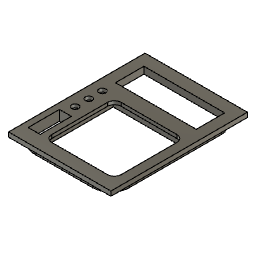
Ferdinant_Deckel v1 (Autodesk Fusion 360 design; units mm, degrees)
Autodesk Fusion 360 part; units mm, degrees
sketch "Skizze1" plane through (0, 0, 0) normal (0, 0, 1) x (1, 0, 0)
  line L0 (-52.263, 59.6389) -> (37.737, 59.6389)
  line L1 (37.737, 59.6389) -> (37.737, -60.3611)
  line L2 (37.737, -60.3611) -> (-52.263, -60.3611)
  line L3 (-52.263, -60.3611) -> (-52.263, 59.6389)
  dimension "d1" = 90
  dimension "d2" = 120
  constraint horizontal L0
  constraint vertical L1
  constraint horizontal L2
  constraint vertical L3
  measures "d1" distance of L0.start L0.end
  measures "d2" distance of L0.end L1.end
extrude "Extrusion1" add sketch "Skizze1" against normal blind 3
extrude "Extrusion2" add 1 faces at (-22.263, 19.6389, 0) along direction (0, 0, 1) blind 1
sketch "Skizze2" plane through (0, 0, 1) normal (0, 0, 1) x (-1, 0, 0)
  line L0 (52.263, 60.3611) -> (-37.737, 60.3611)
  line L1 (-37.737, 60.3611) -> (-37.737, -59.6389)
  line L2 (-37.737, -59.6389) -> (52.263, -59.6389)
  line L3 (52.263, -59.6389) -> (52.263, 60.3611)
  line L4 (25.263, -11.6389) -> (-23.737, -11.6389)
  line L5 (-29.737, -5.6389) -> (-29.737, 43.3611)
  line L6 (-23.737, 49.3611) -> (25.263, 49.3611)
  line L7 (31.263, 43.3611) -> (31.263, -5.6389)
  line L8 (33.263, -12.6389) -> (-31.737, -12.6389)
  line L9 (-31.737, -12.6389) -> (-31.737, 52.3611)
  line L10 (-31.737, 52.3611) -> (33.263, 52.3611)
  line L11 (33.263, 52.3611) -> (33.263, -12.6389)
  line L12 (42.763, -49.1389) -> (-28.237, -49.1389)
  line L13 (-28.237, -49.1389) -> (-28.237, -24.1389)
  line L14 (-28.237, -24.1389) -> (42.763, -24.1389)
  line L15 (42.763, -24.1389) -> (42.763, -49.1389)
  circle A0 centre (42.263, -12.1389) radius 3
  circle A1 centre (42.263, -0.1389) radius 3
  circle A2 centre (42.263, 11.8611) radius 3
  line L16 (47.013, 20.8611) -> (36.513, 20.8611)
  line L17 (36.513, 20.8611) -> (36.513, 48.3611)
  line L18 (36.513, 48.3611) -> (47.013, 48.3611)
  line L19 (47.013, 48.3611) -> (47.013, 20.8611)
  arc A3 (-29.737, -5.6389) -> (-23.737, -11.6389) centre (-23.737, -5.6389) ccw
  arc A4 (25.263, -11.6389) -> (31.263, -5.6389) centre (25.263, -5.6389) ccw
  arc A5 (31.263, 43.3611) -> (25.263, 49.3611) centre (25.263, 43.3611) ccw
  arc A6 (-23.737, 49.3611) -> (-29.737, 43.3611) centre (-23.737, 43.3611) ccw
  point P0 (31.263, -11.6389)
  point P1 (-29.737, -11.6389)
  point P2 (31.263, 49.3611)
  dimension "d7" = 61
  dimension "d8" = 61
  dimension "d10" = 11
  dimension "d11" = 65
  dimension "d12" = 65
  dimension "d13" = 8
  dimension "d19" = 25
  dimension "d20" = 71
  dimension "d23" = 8
  dimension "d24" = 6
  dimension "d25" = 6
  dimension "d26" = 9
  dimension "d28" = 6
  dimension "d29" = 6
  dimension "d30" = 12
  dimension "d31" = 9
  dimension "d32" = 9
  dimension "d33" = 12
  dimension "d34" = 10.5
  dimension "d35" = 27.5
  dimension "d36" = 12
  dimension "d37" = 5.25
  dimension "d62" = 6
  dimension "d63" = 6
  dimension "d82" = 12
  constraint horizontal L4
  constraint vertical L5
  constraint horizontal L6
  constraint vertical L7
  constraint horizontal L8
  constraint vertical L9
  constraint horizontal L10
  constraint vertical L11
  constraint horizontal L12
  constraint vertical L13
  constraint horizontal L14
  constraint vertical L15
  constraint horizontal L16
  constraint vertical L17
  constraint horizontal L18
  constraint vertical L19
  constraint coincident P1 L4
  constraint coincident P1 L5
  constraint tangent L4 A3
  constraint tangent L5 A3
  constraint coincident P0 L4
  constraint coincident P0 L7
  constraint tangent L4 A4
  constraint tangent L7 A4
  constraint coincident P2 L6
  constraint coincident P2 L7
  constraint tangent L6 A5
  constraint tangent L7 A5
  constraint equal A4 A5
  constraint tangent L5 A6
  constraint tangent L6 A6
  constraint equal A4 A6
  measures "d7" distance of P0 P1
  measures "d8" distance of P0 P2
  measures "d10" distance of L0 L6
  measures "d11" distance of L8.start L8.end
  measures "d12" distance of L8.start L10.end
  measures "d13" distance of L0 L10
  measures "d19" distance of L12.start L14.end
  measures "d20" distance of L12.start L12.end
  measures "d23" distance of L1 L5
  measures "d24" distance of L1 L9
  measures "d25" diameter of A0
  measures "d26" distance of L11 A0.centre
  measures "d28" diameter of A1
  measures "d29" diameter of A2
  measures "d30" vertical distance of A0.centre A1.centre
  measures "d31" distance of L11 A1.centre
  measures "d32" distance of L11 A2.centre
  measures "d33" distance of A1.centre A2.centre
  measures "d34" distance of L16.start L16.end
  measures "d35" distance of L16.start L18.end
  measures "d36" distance of L0 L18
  measures "d37" distance of L3 L19
  measures "d62" radius of A3
  measures "d63" radius of A4
  measures "d82" distance of L14 A0.centre
sketch "Skizze3" plane through (0, 0, -3) normal (0, 0, -1) x (1, 0, 0)
  line L0 (37.737, 60.3611) -> (-52.263, 60.3611)
  line L1 (-52.263, 60.3611) -> (-52.263, -59.6389)
  line L2 (-52.263, -59.6389) -> (37.737, -59.6389)
  line L3 (37.737, -59.6389) -> (37.737, 60.3611)
  line L4 (-32.763, 56.8611) -> (18.237, 56.8611)
  line L5 (34.237, 40.8611) -> (34.237, -56.1389)
  line L6 (34.237, -56.1389) -> (-48.763, -56.1389)
  line L7 (-48.763, -56.1389) -> (-48.763, 40.8611)
  arc A0 (34.237, 40.8611) -> (18.237, 56.8611) centre (18.237, 40.8611) ccw
  arc A1 (-32.763, 56.8611) -> (-48.763, 40.8611) centre (-32.763, 40.8611) ccw
  line L8 (-52.263, 0.3611) -> (37.737, 0.3611)
  arc A2 (-48.763, -40.1389) -> (-32.763, -56.1389) centre (-32.763, -40.1389) ccw
  arc A3 (18.237, -56.1389) -> (34.237, -40.1389) centre (18.237, -40.1389) ccw
  dimension "d38" = 3.5
  dimension "d39" = 3.5
  dimension "d40" = 3.5
  dimension "d41" = 3.5
  dimension "d45" = 16
  dimension "d46" = 16
  constraint horizontal L4
  constraint vertical L5
  constraint horizontal L6
  constraint vertical L7
  constraint tangent L4 A0
  constraint tangent L5 A0
  constraint tangent L4 A1
  constraint tangent L7 A1
  constraint midpoint L1 L8.start
  constraint midpoint L3 L8.end
  constraint symmetric L4.end L8 A3.start
  constraint symmetric L5.start L8 A3.end
  constraint symmetric A0 L8 A3
  constraint symmetric L4.start L8 A2.end
  constraint symmetric L7.end L8 A2.start
  constraint symmetric A1 L8 A2
  measures "d38" distance of L1 L7
  measures "d39" distance of L3 L5
  measures "d40" distance of L0 L4
  measures "d41" distance of L2 L6
  measures "d45" radius of A0
  measures "d46" radius of A1
extrude "Extrusion3" add sketch "Skizze3" along normal blind 5 contours L4 L5 L7 A0 A1 L8 | L5 L6 L7 L8 A2 A3
extrude "Extrusion4" cut sketch "Skizze2" against normal blind 9 contours A1
extrude "Extrusion5" cut sketch "Skizze2" against normal blind 9 contours A0 | A2
sketch "Skizze4" plane through (0, 0, -8) normal (0, 0, -1) x (1, 0, 0)
  circle A0 centre (-42.263, -12.1389) radius 3
  circle A1 centre (-42.263, 11.8611) radius 3
  circle A2 centre (-42.263, -0.1389) radius 3
  arc A3 (-48.763, -40.1389) -> (-32.763, -56.1389) centre (-32.763, -40.1389) ccw
  line L0 (-32.763, -56.1389) -> (18.237, -56.1389)
  arc A4 (18.237, -56.1389) -> (34.237, -40.1389) centre (18.237, -40.1389) ccw
  line L1 (34.237, -40.1389) -> (34.237, 40.8611)
  arc A5 (34.237, 40.8611) -> (18.237, 56.8611) centre (18.237, 40.8611) ccw
  line L2 (18.237, 56.8611) -> (-32.763, 56.8611)
  arc A6 (-32.763, 56.8611) -> (-48.763, 40.8611) centre (-32.763, 40.8611) ccw
  line L3 (-48.763, 40.8611) -> (-48.763, -40.1389)
  circle A7 centre (-42.263, 11.8611) radius 4
  circle A8 centre (-42.263, -0.1389) radius 4
  circle A9 centre (-42.263, -12.1389) radius 4
  dimension "d53" = 8
  dimension "d54" = 8
  dimension "d55" = 8
  constraint concentric A1 A7
  constraint concentric A2 A8
  constraint concentric A0 A9
  measures "d53" diameter of A7
  measures "d54" diameter of A8
  measures "d55" diameter of A9
extrude "Extrusion6" cut sketch "Skizze4" against normal blind 6 contours A7 | A8 | A9
extrude "Extrusion7" cut sketch "Skizze2" against normal blind 9 contours L16 L17 L18 L19
extrude "Extrusion8" cut sketch "Skizze2" against normal blind 9 contours L12 L13 L14 L15
extrude "Extrusion9" cut sketch "Skizze2" against normal blind 9 contours L4 L5 L6 L7 A3 A4 A5 A6
sketch "Skizze5" plane through (0, 0, -8) normal (0, 0, -1) x (1, 0, 0)
  line L0 (-25.263, 49.3611) -> (23.737, 49.3611)
  arc A0 (29.737, 43.3611) -> (23.737, 49.3611) centre (23.737, 43.3611) ccw
  line L1 (29.737, 43.3611) -> (29.737, -5.6389)
  arc A1 (23.737, -11.6389) -> (29.737, -5.6389) centre (23.737, -5.6389) ccw
  line L2 (23.737, -11.6389) -> (-25.263, -11.6389)
  arc A2 (-31.263, -5.6389) -> (-25.263, -11.6389) centre (-25.263, -5.6389) ccw
  line L3 (-31.263, -5.6389) -> (-31.263, 43.3611)
  arc A3 (-25.263, 49.3611) -> (-31.263, 43.3611) centre (-25.263, 43.3611) ccw
  line L4 (28.237, -24.1389) -> (28.237, -49.1389)
  line L5 (28.237, -49.1389) -> (-42.763, -49.1389)
  line L6 (-42.763, -49.1389) -> (-42.763, -24.1389)
  line L7 (-42.763, -24.1389) -> (28.237, -24.1389)
  line L8 (-47.013, 20.8611) -> (-47.013, 48.1369)
  arc A4 (-47.013, 48.1369) -> (-48.763, 40.8611) centre (-32.763, 40.8611) ccw
  line L9 (-48.763, 40.8611) -> (-48.763, -40.1389)
  arc A5 (-48.763, -40.1389) -> (-32.763, -56.1389) centre (-32.763, -40.1389) ccw
  line L10 (-32.763, -56.1389) -> (18.237, -56.1389)
  arc A6 (18.237, -56.1389) -> (34.237, -40.1389) centre (18.237, -40.1389) ccw
  line L11 (34.237, -40.1389) -> (34.237, 40.8611)
  arc A7 (34.237, 40.8611) -> (18.237, 56.8611) centre (18.237, 40.8611) ccw
  line L12 (18.237, 56.8611) -> (-32.763, 56.8611)
  arc A8 (-32.763, 56.8611) -> (-46.8963, 48.3611) centre (-32.763, 40.8611) ccw
  line L13 (-46.8963, 48.3611) -> (-36.513, 48.3611)
  line L14 (-36.513, 48.3611) -> (-36.513, 20.8611)
  line L15 (-36.513, 20.8611) -> (-47.013, 20.8611)
  circle A9 centre (-42.263, 11.8611) radius 4
  circle A10 centre (-42.263, -0.1389) radius 4
  circle A11 centre (-42.263, -12.1389) radius 4
  line L16 (32.737, -13.6389) -> (-34.263, -13.6389)
  line L17 (-34.263, -13.6389) -> (-34.263, 53.3611)
  line L18 (-34.263, 53.3611) -> (32.737, 53.3611)
  line L19 (32.737, 53.3611) -> (32.737, -13.6389)
  line L20 (37.737, 60.3611) -> (37.737, -59.6389)
  line L21 (-52.263, 60.3611) -> (37.737, 60.3611)
  dimension "d66" = 67
  dimension "d67" = 67
  dimension "d68" = 5
  dimension "d69" = 7
  constraint horizontal L16
  constraint vertical L17
  constraint horizontal L18
  constraint vertical L19
  measures "d66" distance of L16.start L16.end
  measures "d67" distance of L16.start L18.end
  measures "d68" distance of L19 L20
  measures "d69" distance of L18 L21
extrude "Extrusion10" cut sketch "Skizze5" against normal blind 6 contours A7 L16 L17 L18 L19
sketch "Skizze6" plane through (0, 0, 1) normal (0, 0, 1) x (-1, 0, 0)
  line L0 (42.763, -49.1389) -> (-28.237, -49.1389)
  line L1 (-28.237, -49.1389) -> (-28.237, -24.1389)
sketch "Skizze7" plane through (0, 0, -8) normal (0, 0, -1) x (1, 0, 0)
  line L0 (-34.263, 53.3611) -> (28.2245, 53.3611)
  arc A0 (28.2245, 53.3611) -> (18.237, 56.8611) centre (18.237, 40.8611) ccw
  line L1 (18.237, 56.8611) -> (-32.763, 56.8611)
  arc A1 (-32.763, 56.8611) -> (-46.8963, 48.3611) centre (-32.763, 40.8611) ccw
  line L2 (-46.8963, 48.3611) -> (-36.513, 48.3611)
  line L3 (-36.513, 48.3611) -> (-36.513, 20.8611)
  line L4 (-36.513, 20.8611) -> (-47.013, 20.8611)
  line L5 (-47.013, 20.8611) -> (-47.013, 48.1369)
  arc A2 (-47.013, 48.1369) -> (-48.763, 40.8611) centre (-32.763, 40.8611) ccw
  line L6 (-48.763, 40.8611) -> (-48.763, -40.1389)
  arc A3 (-48.763, -40.1389) -> (-32.763, -56.1389) centre (-32.763, -40.1389) ccw
  line L7 (-32.763, -56.1389) -> (18.237, -56.1389)
  arc A4 (18.237, -56.1389) -> (34.237, -40.1389) centre (18.237, -40.1389) ccw
  line L8 (34.237, -40.1389) -> (34.237, 40.8611)
  arc A5 (34.237, 40.8611) -> (32.737, 47.625) centre (18.237, 40.8611) ccw
  line L9 (32.737, 47.625) -> (32.737, -13.6389)
  line L10 (32.737, -13.6389) -> (-34.263, -13.6389)
  line L11 (-34.263, -13.6389) -> (-34.263, 53.3611)
  line L12 (28.237, -24.1389) -> (28.237, -49.1389)
  line L13 (28.237, -49.1389) -> (-42.763, -49.1389)
  line L14 (-42.763, -49.1389) -> (-42.763, -24.1389)
  line L15 (-42.763, -24.1389) -> (28.237, -24.1389)
  circle A6 centre (-42.263, 11.8611) radius 4
  circle A7 centre (-42.263, -0.1389) radius 4
  circle A8 centre (-42.263, -12.1389) radius 4
  line L16 (33.737, -55.3889) -> (-48.263, -55.3889)
  line L17 (-48.263, -55.3889) -> (-48.263, -17.8889)
  line L18 (-48.263, -17.8889) -> (33.737, -17.8889)
  line L19 (33.737, -17.8889) -> (33.737, -55.3889)
  line L20 (-42.763, -49.1389) -> (28.237, -49.1389)
  line L21 (28.237, -49.1389) -> (28.237, -24.1389)
  dimension "d76" = 82
  dimension "d77" = 37.5
  dimension "d78" = 6.25
  dimension "d79" = 5.5
  constraint horizontal L16
  constraint vertical L17
  constraint horizontal L18
  constraint vertical L19
  measures "d76" distance of L16.start L16.end
  measures "d77" distance of L16.start L18.end
  measures "d78" distance of L16 L20
  measures "d79" distance of L19 L21
extrude "Extrusion11" cut sketch "Skizze7" against normal blind 3 contours A4 L16 L19 | A3 A4 L16 L17 L18 L19 | A3 L16 L17
